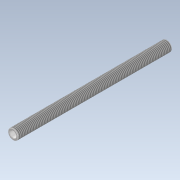
# Autodesk Inventor part: eje manzana
Saved by Autodesk Inventor 2021 (Build 250183000, 183)
## iProperties
Created: 2021-04-24
Part Number: eje manzana
Material: Genérico
Document SubType Name: Modeling
Designer: j2seb
Density: 1 g/cm^3
Appearance: Valor por defecto
Author: j2seb
Autodesk Inventor part; units mm, degrees
ref_plane "YZ Plane" through (0, 0, 0) normal (1, 0, 0) x (0, 1, 0)
ref_plane "XZ Plane" through (0, 0, 0) normal (0, 1, 0) x (-1, 0, 0)
ref_plane "XY Plane" through (0, 0, 0) normal (0, 0, 1) x (1, 0, 0)
sketch "Boceto1" plane through (0, 0, 0) normal (1, 0, 0) x (0, 1, 0)
  line L0 (0, 75) -> (0, -75)
  line L1 (3, 75) -> (5, 75)
  line L2 (5, 75) -> (5, -75)
  line L3 (5, -75) -> (3, -75)
  line L4 (3, -75) -> (3, 75)
  point P0 (0, 0)
  point P1 (0, 0)
  dimension "d0" = 150
  dimension "d1" = 10
  dimension "d3" = 2
  constraints: 10 end point, 2 horizontal alignment, 2 parallel, 1 coincident, 1 horizontal, 1 midpoint, 1 perpendicular, 1 vertical
  measures "d0" distance of L0.start L0.end
  measures "d1" diameter of L2 L0
  measures "d3" distance between parallel lines of L4 L2
revolve "Revolución1" add sketch "Boceto1" angle 360 about axis through (0, 0, 75) along (0, 0, -1)
thread "Rosca1" size "M10x1.5" class "6g" standard "ANSI Metric M Profile" full length
chamfer "Chaflán1" distance 0.5 angle 45 4 edges at (0, -3, 75) (0, -5, 75) (0, -5, -75) (0, -3, -75)
